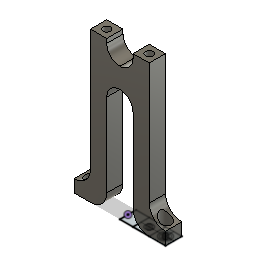
_Annikas IMU (probably not interference but whatev.c6cc2b10-ba41-4698-b681-40151d34f9de (Autodesk Fusion 360 design; units mm, degrees)
Autodesk Fusion 360 part; units mm, degrees
sketch "Sketch1" plane through (0, 0, 0) normal (0, 1, 0) x (1, 0, 0)
  circle A0 centre (15, 0) radius 1.65
  circle A1 centre (15, 0) radius 2.25
  line L0 (0, -3.25) -> (0, 3.25)
  line L1 (0, 3.25) -> (18.25, 3.25)
  line L2 (18.25, 3.25) -> (18.25, -3.25)
  line L3 (18.25, -3.25) -> (0, -3.25)
  line L4 (15, 0) -> (15, 2.25) construction
  line L5 (15, 2.25) -> (15, 3.25) construction
  line L6 (15, 0) -> (17.25, 0) construction
  line L7 (17.25, 0) -> (18.25, 0) construction
  line L8 (11.75, 3.25) -> (11.75, -3.25)
  line L9 (5.25, 3.25) -> (5.25, -3.25)
  line L10 (5.25, -3.25) -> (11.75, -3.25) construction
  circle A2 centre (8.5, 0) radius 1.5
  line L11 (8.5, 0) -> (11.75, 0) construction
  line L12 (8.5, 0) -> (5.25, 0) construction
  line L13 (11.75, 0) -> (12.75, 0) construction
  dimension "d1" = 3.3
  dimension "d3" = 4.5
  dimension "d4" = 15
  dimension "d15" = 8.5
  dimension "d16" = 3
  constraint concentric A0 A1
  constraint vertical L0
  constraint perpendicular L0 L1
  constraint perpendicular L1 L2
  constraint perpendicular L0 L3
  constraint midpoint origin L0
  constraint coincident A0.centre A1.centre
  constraint coincident A1 L4.end
  constraint vertical L4
  constraint coincident L1 L5.end
  constraint perpendicular L1 L5
  constraint coincident A1 L6.end
  constraint perpendicular L4 L6
  constraint midpoint L2 L7.end
  constraint perpendicular L2 L7
  constraint equal L5 L7
  constraint coincident L1 L8.start
  constraint coincident L3 L8.end
  constraint perpendicular L3 L8
  constraint coincident L1 L9.start
  constraint coincident L3 L9.end
  constraint perpendicular L3 L9
  constraint equal L9 L10
  constraint coincident A2.centre L11.start
  constraint midpoint L8 L11.end
  constraint midpoint L9 L12.end
  constraint equal L11 L12
  constraint horizontal L11
  constraint coincident A1 L13.end
  constraint perpendicular L8 L13
  constraint equal L7 L13
  measures "d1" diameter of A0
  measures "d3" diameter of A1
  measures "d4" distance of origin A0.centre
  measures "d15" distance of L0 A2.centre
  measures "d16" diameter of A2
extrude "Extrude1" add sketch "Sketch1" along normal blind 5 contours A0 | A1 | L1 L2 L3 L8
extrude "Extrude2" add sketch "Sketch1" along normal blind 2 contours A1
extrude "Extrude3" add sketch "Sketch1" along normal blind 60 contours L1 L3 L8 L9 | A2
extrude "Extrude4" add sketch "Sketch1" along normal blind 53 and the other way blind -45 contours L0 L1 L3 L9
extrude "Extrude5" cut sketch "Sketch1" along normal blind 60 and the other way blind -52 contours A2
fillet "Fillet1" radius 5.3 2 edges at (5.25, 53, 0) (5.25, 45, 0)
fillet "Fillet1" radius 6.5 2 edges at (11.75, 5, 0) (5.25, 0, 0)
extrude "Extrude6" cut sketch "Sketch1" along normal blind 18 contours A0
extrude "Extrude7" cut sketch "Sketch1" along normal blind 16.5 and the other way blind -2 contours A1
mirror "Mirror1" about plane through (0, 45, 3.25) normal (-1, 0, 0) of bodies 1 merged
equation "d15 = ( 17 / 2 ) * 1 mm"
